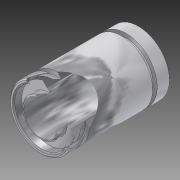
# Autodesk Inventor part: bearing
Saved by Autodesk Inventor 2014 SP1 (Build 180222100, 222)
## iProperties
Created: 2017-07-23
Part Number: bearing
Material: Типовые
Document SubType Name: Modeling
Designer: Stepan
Density: 1 g/cm^3
Appearance: Алюминий — полированный
Author: Stepan
Autodesk Inventor part; units mm, degrees
ref_plane "YZ Plane" through (0, 0, 0) normal (1, 0, 0) x (0, 1, 0)
ref_plane "XZ Plane" through (0, 0, 0) normal (0, 1, 0) x (-1, 0, 0)
ref_plane "XY Plane" through (0, 0, 0) normal (0, 0, 1) x (1, 0, 0)
sketch "Эскиз1" plane through (0, 0, 0) normal (0, 0, 1) x (1, 0, 0)
  line L0 (0, 0) -> (0, 24) construction
  line L1 (0, 24) -> (4, 24) construction
  line L2 (4, 24) -> (4, 0)
  line L3 (4, 24) -> (7.5, 24)
  line L4 (7.5, 24) -> (7.5, 20.75)
  line L5 (7.5, 20.75) -> (6.5, 20.75)
  line L6 (6.5, 20.75) -> (6.5, 19.65)
  line L7 (6.5, 19.65) -> (7.5, 19.65)
  line L8 (7.5, 19.65) -> (7.5, 4.35)
  line L9 (7.5, 4.35) -> (6.5, 4.35)
  line L10 (6.5, 4.35) -> (6.5, 3.25)
  line L11 (6.5, 3.25) -> (7.5, 3.25)
  line L12 (7.5, 3.25) -> (7.5, 0)
  line L13 (7.5, 0) -> (4, 0)
  dimension "d0" = 24
  dimension "d1" = 4
  dimension "d3" = 3.5
  dimension "d4" = 3.25
  dimension "d5" = 1
  dimension "d6" = 1.1
  dimension "d7" = 15.3
  dimension "d8" = 1
  dimension "d9" = 1.1
  constraints: 28 end point, 8 perpendicular, 3 parallel, 2 point on line, 1 collinear, 1 vertical
  measures "d0" distance of L0.start L0.end
  measures "d1" distance of L0.end L1.end
  measures "d3" distance of L1.end L3.end
  measures "d4" distance of L3.end L4.end
  measures "d5" distance of L4.end L5.end
  measures "d6" distance of L5.end L6.end
  measures "d7" distance of L7.end L8.end
  measures "d8" distance of L8.end L9.end
  measures "d9" distance of L9.end L10.end
revolve "Вращение1" add sketch "Эскиз1" angle 360 about axis through (0, 0, 0) along (0, 1, 0)
chamfer "Фаска1" distance 0.3 angle 45 2 edges at (-7.5, 24, 0) (-7.5, 0, 0)
sketch "Эскиз2" plane through (0, 24, 0) normal (0, 1, 0) x (1, 0, 0)
  circle A0 centre (0, 0) radius 4 projected
  circle A1 centre (0, 0) radius 7.2 projected
  circle A2 centre (0, 0) radius 6.5
  dimension "d14" = 13
  constraints: 1 centre point, 1 coincident
  measures "d14" diameter of A2
extrude "Выдавливание1" cut sketch "Эскиз2" against normal blind 2 contours A2
chamfer "Фаска2" distance 0.3 angle 45 1 edges at (-6.5, 24, 0)
sketch "Эскиз4" plane through (0, 0, 0) normal (0, -1, 0) x (1, 0, 0)
  circle A0 centre (0, 0) radius 4 projected
  circle A1 centre (0, 0) radius 7.2 projected
  circle A2 centre (0, 0) radius 6.5
  dimension "d27" = 13
  constraints: 1 centre point, 1 coincident
  measures "d27" diameter of A2
extrude "Выдавливание3" cut sketch "Эскиз4" against normal blind 2 contours A2
chamfer "Фаска4" distance 0.3 angle 45 1 edges at (-6.5, 0, 0)
